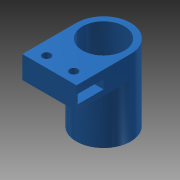
# Autodesk Inventor part: paint holder
Saved by Autodesk Inventor 2013 (Build 170138000, 138)
## iProperties
Created: 2017-01-26
Part Number: paint holder
Material: Generic
Document SubType Name: Modeling
Designer: Herman de Vries
Density: 1 g/cm^3
Author: Herman de Vries
Autodesk Inventor part; units mm, degrees
ref_plane "YZ Plane" through (0, 0, 0) normal (1, 0, 0) x (0, 1, 0)
ref_plane "XZ Plane" through (0, 0, 0) normal (0, 1, 0) x (-1, 0, 0)
sketch "Sketch1" plane through (0, 0, 0) normal (0, 0, 1) x (1, 0, 0)
  line L0 (0, 0) -> (20, 0)
  line L1 (20, 0) -> (20, 20)
  line L2 (10, 30) -> (10, 30)
  line L3 (0, 20) -> (0, 0)
  circle A0 centre (10, 20) radius 7.75
  circle A1 centre (5, 4) radius 1.5
  circle A2 centre (15, 4) radius 1.5
  arc A3 (10, 30) -> (0, 20) centre (10, 20) ccw
  arc A4 (20, 20) -> (10, 30) centre (10, 20) ccw
  point P0 (20, 30)
  point P1 (0, 30)
  dimension "d0" = 20
  dimension "d1" = 30
  dimension "d4" = 15.5
  dimension "d5" = 10
  dimension "d6" = 3
  dimension "d7" = 3
  dimension "d8" = 4
  dimension "d9" = 10
  dimension "d10" = 5
  dimension "d11" = 5
  dimension "d20" = 10
  constraints: 8 end point, 5 centre point, 4 point on circle, 4 point on line, 4 tangent, 2 parallel, 1 concentric, 1 horizontal, 1 horizontal alignment, 1 midpoint, 1 perpendicular, 1 vertical alignment
  measures "d0" distance of point (0, 30) point (20, 30)
  measures "d1" distance of point (20, 30) L0.end
  measures "d4" diameter of A0
  measures "d5" distance from line of L2 A0.centre
  measures "d6" diameter of A1
  measures "d7" diameter of A2
  measures "d8" distance from line of L0 A1.centre
  measures "d9" distance of A2.centre A1.centre
  measures "d10" distance from line of L3 A1.centre
  measures "d11" distance from line of L1 A2.centre
  measures "d20" radius of A3
extrude "Extrusion1" add sketch "Sketch1" along normal blind 3
sketch "Sketch2" plane through (0, 0, 0) normal (0, 0, -1) x (-1, 0, 0)
  circle A0 centre (-10, 20) radius 7.75 projected
  circle A1 centre (-10, 20) radius 10
  arc A2 (0, 20) -> (-20, 20) centre (-10, 20) ccw projected
  point P0 (0, 0)
  constraints: 1 coincident, 1 horizontal alignment, 3 other
extrude "Extrusion2" add sketch "Sketch2" along normal blind 25
sketch "Sketch6" plane through (0, 0, 0) normal (0, -1, 0) x (1, 0, 0)
  line L0 (0, 0) -> (-1.6294, 0)
  line L1 (-1.6294, 0) -> (-1.6294, -3.3)
  line L2 (-1.6294, -3.3) -> (0, -3.3)
  line L3 (0, -3.3) -> (0, 0)
  dimension "d25" = 3.3
  constraints: 8 end point, 2 parallel, 1 horizontal, 1 perpendicular
  measures "d25" distance of L1.end L0.end
ref_plane "Work Plane1" through (-1.6294, 0, -3.3) normal (0, 0, -1) x (-1, 0, 0)
ref_plane "Work Plane2" through (-1.6294, 0, -3.3) normal (0, 0, -1) x (-1, 0, 0)
sketch "Sketch3" plane through (-1.6294, 0, -3.3) normal (0, 0, -1) x (-1, 0, 0)
  line L0 (-1.6294, 0) -> (-21.6294, 0) projected
  line L1 (-1.6294, 20) -> (-1.6294, 0) projected
  arc A0 (-21.6294, 20) -> (-1.6294, 20) centre (-11.6294, 20) ccw projected
  line L2 (-21.6294, 0) -> (-21.6294, 20) projected
  circle A1 centre (-6.6294, 4) radius 1.5 projected
  circle A2 centre (-16.6294, 4) radius 1.5 projected
extrude "Extrusion3" add sketch "Sketch3" along normal blind 2
sketch "Sketch4" plane through (0, 0, 0) normal (0, 0, -1) x (-1, 0, 0)
  circle A0 centre (-10, 20) radius 10 projected
  line L0 (-20, 10) -> (0, 10)
  line L1 (-20, 10) -> (-20, 20)
  line L2 (0, 10) -> (0, 20)
  line L3 (-20, 0) -> (0, 0)
  line L4 (0, 0) -> (0, 0.4)
  line L5 (0, 0.4) -> (-20, 0.4)
  line L6 (-20, 0.4) -> (-20, 0)
  line L7 (-20, 0) -> (-20, 20) projected
  line L8 (0, 20) -> (0, 0) projected
  dimension "d21" = 0.4
  constraints: 14 end point, 3 parallel, 3 tangent, 2 point on circle, 2 point on line, 1 horizontal, 1 perpendicular
  measures "d21" distance of L4.end L3.end
extrude "Extrusion4" add sketch "Sketch4" along normal up to surface (3.3 mm away) contours L2 L0 A0 | A0 L0 L1 | L4 L3 L6 L5
sketch "Sketch5" plane through (-1.6294, 0, -3.3) normal (0, 0, 1) x (1, 0, 0)
  circle A0 centre (16.6294, 4) radius 1.5 projected
  circle A1 centre (6.6294, 4) radius 1.5 projected
  point P0 (1.6294, 0)
extrude "Extrusion5" add sketch "Sketch5" against normal blind 0.2
equation "\"d10\" = d11"
body "Solid1"
